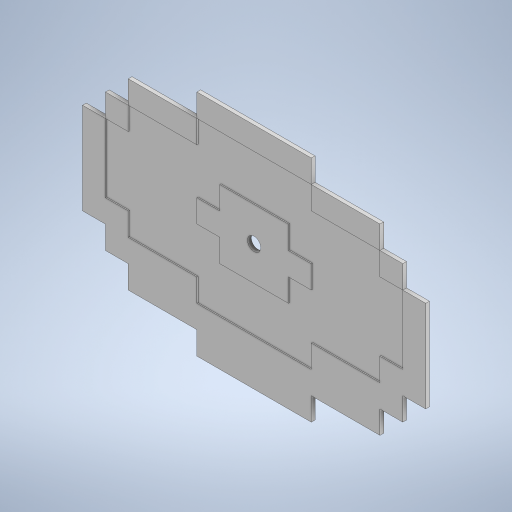
# Autodesk Inventor part: horizantal cut norm center
Saved by Autodesk Inventor 2024 (Build 280153000, 153)
## iProperties
Created: 2024-02-02
Part Number: horizantal cut norm center
Material: Generic
Document SubType Name: Modeling
Designer: newic
Density: 1 g/cm^3
Appearance: Default
Author: newic
Autodesk Inventor part; units mm, degrees
ref_plane "YZ Plane" through (0, 0, 0) normal (1, 0, 0) x (0, 1, 0)
ref_plane "XZ Plane" through (0, 0, 0) normal (0, 1, 0) x (-1, 0, 0)
ref_plane "XY Plane" through (0, 0, 0) normal (0, 0, 1) x (1, 0, 0)
sketch "Sketch1" plane through (0, 0, 0) normal (0, 0, 1) x (1, 0, 0)
  circle A0 centre (0, 0) radius 152.4
  circle A1 centre (0, 0) radius 5.5
  dimension "d0" = 304.8
  dimension "d1" = 11
  constraints: 2 centre point, 2 coincident
  measures "d0" diameter of A0
  measures "d1" diameter of A1
extrude "Extrusion1" add sketch "Sketch1" along normal blind 2.2
fillet "Fillet1" radius 1.1 2 edges at (-152.4, 0, 0) (-152.4, 0, 2.2)
sketch "Sketch2" plane through (0, 0, 2.2) normal (0, 0, 1) x (1, 0, 0)
  line L0 (206.2137, 42.4617) -> (289.822, 42.4617) construction
  line L1 (289.822, 42.4617) -> (289.822, -13.3654) construction
  line L2 (289.822, -13.3654) -> (206.2137, -13.3654) construction
  line L3 (206.2137, -13.3654) -> (206.2137, 42.4617) construction
  line L4 (9.525, 9.525) -> (-9.525, 9.525)
  line L5 (-9.525, 9.525) -> (-9.525, -9.525)
  line L6 (-9.525, -9.525) -> (9.525, -9.525)
  line L7 (9.525, -9.525) -> (9.525, 9.525)
  line L8 (-123.825, 28.575) -> (-104.775, 28.575)
  line L9 (-85.725, 28.575) -> (-66.675, 28.575)
  line L10 (-85.725, 28.575) -> (-104.775, 28.575)
  line L11 (-9.525, 28.575) -> (-28.575, 28.575)
  line L12 (-47.625, 28.575) -> (-28.575, 28.575)
  line L13 (-47.625, 28.575) -> (-66.675, 28.575)
  line L14 (-9.525, 9.525) -> (-9.525, 28.575)
  line L15 (-9.525, 28.575) -> (9.525, 28.575)
  line L16 (9.525, 28.575) -> (9.525, 9.525)
  line L17 (-9.525, -28.575) -> (-9.525, -9.525)
  line L18 (9.525, -9.525) -> (9.525, -28.575)
  line L19 (-123.825, -47.625) -> (-142.875, -47.625)
  line L20 (-123.825, -47.625) -> (-104.775, -47.625)
  line L21 (-85.725, -47.625) -> (-104.775, -47.625)
  line L22 (-85.725, -47.625) -> (-66.675, -47.625)
  line L23 (-47.625, -47.625) -> (-66.675, -47.625)
  line L24 (-47.625, -47.625) -> (-28.575, -47.625)
  line L25 (-9.525, -47.625) -> (-28.575, -47.625)
  line L26 (-9.525, -28.575) -> (-9.525, -47.625)
  line L27 (9.525, -47.625) -> (9.525, -28.575)
  line L28 (142.875, 28.575) -> (123.825, 28.575)
  line L29 (104.775, 28.575) -> (123.825, 28.575)
  line L30 (104.775, 28.575) -> (85.725, 28.575)
  line L31 (66.675, 28.575) -> (85.725, 28.575)
  line L32 (66.675, 28.575) -> (47.625, 28.575)
  line L33 (28.575, 28.575) -> (47.625, 28.575)
  line L34 (28.575, 28.575) -> (9.525, 28.575)
  line L35 (104.775, -47.625) -> (123.825, -47.625)
  line L36 (104.775, -47.625) -> (85.725, -47.625)
  line L37 (142.875, -47.625) -> (123.825, -47.625)
  line L38 (66.675, -47.625) -> (85.725, -47.625)
  line L39 (66.675, -47.625) -> (47.625, -47.625)
  line L40 (28.575, -47.625) -> (47.625, -47.625)
  line L41 (28.575, -47.625) -> (9.525, -47.625)
  line L42 (0, 9.525) -> (0, -9.525)
  line L43 (-9.525, 0) -> (9.525, 0)
  line L44 (0, 0) -> (-4.1012, 3.8959)
  line L45 (-142.875, 28.575) -> (-123.825, 28.575)
  line L46 (-123.825, 28.575) -> (-123.825, 9.525)
  line L47 (-123.825, 9.525) -> (-142.875, 9.525)
  line L48 (-142.875, 9.525) -> (-142.875, 28.575)
  line L49 (-142.875, -9.525) -> (-123.825, -9.525)
  line L50 (-123.825, -9.525) -> (-123.825, 9.525)
  line L51 (-142.875, 9.525) -> (-142.875, -9.525)
  line L52 (-123.825, -47.625) -> (-123.825, -28.575)
  line L53 (-123.825, -28.575) -> (-142.875, -28.575)
  line L54 (-142.875, -28.575) -> (-142.875, -47.625)
  line L55 (-123.825, -9.525) -> (-123.825, -28.575)
  line L56 (-142.875, -28.575) -> (-142.875, -9.525)
  line L57 (123.825, -47.625) -> (142.875, -47.625)
  line L58 (142.875, 28.575) -> (123.825, 28.575)
  line L59 (123.825, 28.575) -> (123.825, 9.525)
  line L60 (123.825, 9.525) -> (142.875, 9.525)
  line L61 (142.875, 9.525) -> (142.875, 28.575)
  line L62 (123.825, -9.525) -> (123.825, 9.525)
  line L63 (142.875, -9.525) -> (123.825, -9.525)
  line L64 (142.875, 9.525) -> (142.875, -9.525)
  line L65 (123.825, -9.525) -> (123.825, -28.575)
  line L66 (123.825, -47.625) -> (123.825, -28.575)
  line L67 (142.875, -28.575) -> (142.875, -9.525)
  line L68 (123.825, -28.575) -> (142.875, -28.575)
  line L69 (142.875, -28.575) -> (142.875, -47.625)
  line L70 (-123.825, 28.575) -> (-104.775, 28.575)
  line L71 (-104.775, 28.575) -> (-104.775, 47.625)
  line L72 (-104.775, 47.625) -> (-123.825, 47.625)
  line L73 (-123.825, 47.625) -> (-123.825, 28.575)
  line L74 (123.825, 28.575) -> (104.775, 28.575)
  line L75 (104.775, 28.575) -> (104.775, 47.625)
  line L76 (104.775, 47.625) -> (123.825, 47.625)
  line L77 (123.825, 47.625) -> (123.825, 28.575)
  line L78 (123.825, -47.625) -> (104.775, -47.625)
  line L79 (104.775, -47.625) -> (104.775, -66.675)
  line L80 (104.775, -66.675) -> (123.825, -66.675)
  line L81 (123.825, -66.675) -> (123.825, -47.625)
  line L82 (-123.825, -47.625) -> (-104.775, -47.625)
  line L83 (-104.775, -47.625) -> (-104.775, -66.675)
  line L84 (-104.775, -66.675) -> (-123.825, -66.675)
  line L85 (-123.825, -66.675) -> (-123.825, -47.625)
  line L86 (104.775, -66.675) -> (85.725, -66.675)
  line L87 (85.725, -66.675) -> (85.725, -85.725)
  line L88 (85.725, -85.725) -> (104.775, -85.725)
  line L89 (104.775, -85.725) -> (104.775, -66.675)
  line L90 (-104.775, -66.675) -> (-85.725, -66.675)
  line L91 (-85.725, -66.675) -> (-85.725, -85.725)
  line L92 (-85.725, -85.725) -> (-104.775, -85.725)
  line L93 (-104.775, -85.725) -> (-104.775, -66.675)
  line L94 (-66.675, -66.675) -> (-85.725, -66.675)
  line L95 (-85.725, -85.725) -> (-66.675, -85.725)
  line L96 (-66.675, -85.725) -> (-66.675, -66.675)
  line L97 (-47.625, -66.675) -> (-47.625, -85.725)
  line L98 (-47.625, -85.725) -> (-66.675, -85.725)
  line L99 (-66.675, -66.675) -> (-47.625, -66.675)
  line L100 (66.675, -66.675) -> (85.725, -66.675)
  line L101 (85.725, -85.725) -> (66.675, -85.725)
  line L102 (66.675, -85.725) -> (66.675, -66.675)
  line L103 (47.625, -66.675) -> (47.625, -85.725)
  line L104 (66.675, -66.675) -> (47.625, -66.675)
  line L105 (47.625, -85.725) -> (66.675, -85.725)
  line L106 (-47.625, -85.725) -> (-28.575, -85.725)
  line L107 (-28.575, -85.725) -> (-28.575, -104.775)
  line L108 (-28.575, -104.775) -> (-47.625, -104.775)
  line L109 (-47.625, -104.775) -> (-47.625, -85.725)
  line L110 (-9.525, -85.725) -> (-28.575, -85.725)
  line L111 (-28.575, -104.775) -> (-9.525, -104.775)
  line L112 (-9.525, -104.775) -> (-9.525, -85.725)
  line L113 (28.575, -85.725) -> (9.525, -85.725)
  line L114 (9.525, -85.725) -> (9.525, -104.775)
  line L115 (9.525, -104.775) -> (28.575, -104.775)
  line L116 (28.575, -104.775) -> (28.575, -85.725)
  line L117 (-9.525, -85.725) -> (9.525, -85.725)
  line L118 (9.525, -104.775) -> (-9.525, -104.775)
  line L119 (28.575, -85.725) -> (47.625, -85.725)
  line L120 (47.625, -85.725) -> (47.625, -104.775)
  line L121 (47.625, -104.775) -> (28.575, -104.775)
  line L122 (-104.775, 47.625) -> (-85.725, 47.625)
  line L123 (-85.725, 47.625) -> (-85.725, 66.675)
  line L124 (-85.725, 66.675) -> (-104.775, 66.675)
  line L125 (-104.775, 66.675) -> (-104.775, 47.625)
  line L126 (104.775, 47.625) -> (85.725, 47.625)
  line L127 (85.725, 47.625) -> (85.725, 66.675)
  line L128 (85.725, 66.675) -> (104.775, 66.675)
  line L129 (104.775, 66.675) -> (104.775, 47.625)
  line L130 (-66.675, 47.625) -> (-85.725, 47.625)
  line L131 (-85.725, 66.675) -> (-66.675, 66.675)
  line L132 (-66.675, 66.675) -> (-66.675, 47.625)
  line L133 (-47.625, 47.625) -> (-47.625, 66.675)
  line L134 (-66.675, 47.625) -> (-47.625, 47.625)
  line L135 (-47.625, 66.675) -> (-66.675, 66.675)
  line L136 (66.675, 47.625) -> (85.725, 47.625)
  line L137 (85.725, 66.675) -> (66.675, 66.675)
  line L138 (66.675, 66.675) -> (66.675, 47.625)
  line L139 (47.625, 47.625) -> (47.625, 66.675)
  line L140 (66.675, 47.625) -> (47.625, 47.625)
  line L141 (47.625, 66.675) -> (66.675, 66.675)
  line L142 (-47.625, 66.675) -> (-28.575, 66.675)
  line L143 (-28.575, 66.675) -> (-28.575, 85.725)
  line L144 (-28.575, 85.725) -> (-47.625, 85.725)
  line L145 (-47.625, 85.725) -> (-47.625, 66.675)
  line L146 (47.625, 66.675) -> (28.575, 66.675)
  line L147 (28.575, 66.675) -> (28.575, 85.725)
  line L148 (28.575, 85.725) -> (47.625, 85.725)
  line L149 (47.625, 85.725) -> (47.625, 66.675)
  line L150 (-9.525, 66.675) -> (-28.575, 66.675)
  line L151 (-28.575, 85.725) -> (-9.525, 85.725)
  line L152 (-9.525, 85.725) -> (-9.525, 66.675)
  line L153 (28.575, 66.675) -> (9.525, 66.675)
  line L154 (9.525, 66.675) -> (9.525, 85.725)
  line L155 (9.525, 85.725) -> (28.575, 85.725)
  line L156 (28.575, 85.725) -> (28.575, 66.675)
  line L157 (-9.525, 66.675) -> (9.525, 66.675)
  line L158 (9.525, 85.725) -> (-9.525, 85.725)
  circle A0 centre (0, 0) radius 225.16
  point P0 (-123.825, -9.525)
  point P1 (-123.825, -47.625)
  point P2 (123.825, -9.525)
  dimension "d22" = 19.05
  dimension "d23" = 19.05
  dimension "d29" = 19.05
  dimension "d30" = 19.05
  dimension "d31" = 19.05
  dimension "d32" = 19.05
  dimension "d33" = 19.05
  dimension "d34" = 19.05
  dimension "d35" = 19.05
  dimension "d36" = 19.05
  dimension "d39" = 19.05
  dimension "d40" = 19.05
  dimension "d45" = 19.05
  dimension "d46" = 19.05
  dimension "d50" = 19.05
  dimension "d51" = 19.05
  dimension "d52" = 19.05
  dimension "d53" = 19.05
  dimension "d58" = 19.05
  dimension "d59" = 19.05
  dimension "d60" = 19.05
  dimension "d61" = 19.05
  constraints: 310 end point, 60 symmetric about line, 24 parallel, 12 horizontal, 12 perpendicular, 5 midpoint, 1 centre point, 1 coincident, 2 other
  measures "d22" distance of L46.end L47.end
  measures "d23" distance of L45.end L46.end
  measures "d29" distance of L72.end L71.end
  measures "d30" distance of L71.end L70.end
  measures "d31" distance of L75.end L76.end
  measures "d32" distance of L74.end L75.end
  measures "d33" distance of L80.end L79.end
  measures "d34" distance of L79.end L78.end
  measures "d35" distance of L83.end L84.end
  measures "d36" distance of L82.end L83.end
  measures "d39" distance of L91.end L92.end
  measures "d40" distance of L90.end L91.end
  measures "d45" distance of L107.end L108.end
  measures "d46" distance of L106.end L107.end
  measures "d50" distance of L124.end L123.end
  measures "d51" distance of L123.end L122.end
  measures "d52" distance of L127.end L128.end
  measures "d53" distance of L126.end L127.end
  measures "d58" distance of L144.end L143.end
  measures "d59" distance of L143.end L142.end
  measures "d60" distance of L147.end L148.end
  measures "d61" distance of L146.end L147.end
extrude "Extrusion2" cut sketch "Sketch2" against normal blind 25.4
sketch "Sketch3" plane through (0, 0, 2.2) normal (0, 0, 1) x (1, 0, 0)
  line L0 (194.8549, 38.1597) -> (278.4632, 38.1597) construction
  line L1 (278.4632, 38.1597) -> (278.4632, -17.6674) construction
  line L2 (278.4632, -17.6674) -> (194.8549, -17.6674) construction
  line L3 (194.8549, -17.6674) -> (194.8549, 38.1597) construction
  line L4 (-123.825, 28.575) -> (-104.775, 28.575)
  line L5 (-123.825, -47.625) -> (-142.875, -47.625)
  line L6 (104.775, 28.575) -> (123.825, 28.575)
  line L7 (142.875, 28.575) -> (123.825, 28.575)
  line L8 (142.875, -47.625) -> (123.825, -47.625)
  line L9 (-142.875, 28.575) -> (-123.825, 28.575)
  line L10 (-123.825, 28.575) -> (-123.825, 9.525)
  line L11 (-142.875, 9.525) -> (-142.875, 28.575)
  line L12 (-123.825, -9.525) -> (-123.825, 9.525)
  line L13 (-142.875, 9.525) -> (-142.875, -9.525)
  line L14 (-123.825, -9.525) -> (-123.825, -28.575)
  line L15 (-142.875, -28.575) -> (-142.875, -9.525)
  line L16 (-142.875, -28.575) -> (-142.875, -47.625)
  line L17 (123.825, -9.525) -> (123.825, 9.525)
  line L18 (142.875, 9.525) -> (142.875, -9.525)
  line L19 (123.825, 28.575) -> (123.825, 9.525)
  line L20 (142.875, 9.525) -> (142.875, 28.575)
  line L21 (142.875, 28.575) -> (123.825, 28.575)
  line L22 (123.825, -9.525) -> (123.825, -28.575)
  line L23 (142.875, -28.575) -> (142.875, -9.525)
  line L24 (142.875, -28.575) -> (142.875, -47.625)
  line L25 (123.825, -47.625) -> (142.875, -47.625)
  line L26 (-123.825, 28.575) -> (-104.775, 28.575)
  line L27 (-104.775, 28.575) -> (-104.775, 47.625)
  line L28 (-104.775, 47.625) -> (-123.825, 47.625)
  line L29 (-123.825, 47.625) -> (-123.825, 28.575)
  line L30 (123.825, 28.575) -> (104.775, 28.575)
  line L31 (104.775, 28.575) -> (104.775, 47.625)
  line L32 (104.775, 47.625) -> (123.825, 47.625)
  line L33 (123.825, 47.625) -> (123.825, 28.575)
  line L34 (104.775, -66.675) -> (123.825, -66.675)
  line L35 (123.825, -66.675) -> (123.825, -47.625)
  line L36 (-104.775, -66.675) -> (-123.825, -66.675)
  line L37 (-123.825, -66.675) -> (-123.825, -47.625)
  line L38 (85.725, -85.725) -> (104.775, -85.725)
  line L39 (104.775, -85.725) -> (104.775, -66.675)
  line L40 (-85.725, -85.725) -> (-104.775, -85.725)
  line L41 (-104.775, -85.725) -> (-104.775, -66.675)
  line L42 (-85.725, -85.725) -> (-66.675, -85.725)
  line L43 (-47.625, -85.725) -> (-66.675, -85.725)
  line L44 (85.725, -85.725) -> (66.675, -85.725)
  line L45 (47.625, -85.725) -> (66.675, -85.725)
  line L46 (-28.575, -104.775) -> (-47.625, -104.775)
  line L47 (-47.625, -104.775) -> (-47.625, -85.725)
  line L48 (-28.575, -104.775) -> (-9.525, -104.775)
  line L49 (9.525, -104.775) -> (-9.525, -104.775)
  line L50 (9.525, -104.775) -> (28.575, -104.775)
  line L51 (47.625, -85.725) -> (47.625, -104.775)
  line L52 (47.625, -104.775) -> (28.575, -104.775)
  line L53 (-104.775, 47.625) -> (-85.725, 47.625)
  line L54 (-85.725, 66.675) -> (-104.775, 66.675)
  line L55 (-104.775, 66.675) -> (-104.775, 47.625)
  line L56 (104.775, 66.675) -> (104.775, 47.625)
  line L57 (-66.675, 47.625) -> (-85.725, 47.625)
  line L58 (-85.725, 66.675) -> (-66.675, 66.675)
  line L59 (-66.675, 47.625) -> (-47.625, 47.625)
  line L60 (-47.625, 66.675) -> (-66.675, 66.675)
  line L61 (-47.625, 47.625) -> (-47.625, 66.675)
  line L62 (-47.625, 85.725) -> (-47.625, 66.675)
  circle A0 centre (0, 0) radius 225.16
  line L63 (-47.625, 85.725) -> (47.625, 85.725)
  line L64 (47.625, 85.725) -> (47.625, 66.675)
  line L65 (47.625, 66.675) -> (-47.625, 66.675)
  line L66 (-47.625, 66.675) -> (-47.625, 85.725)
  line L67 (47.625, 66.675) -> (104.775, 66.675)
  line L68 (104.775, 66.675) -> (104.775, 47.625)
  line L69 (104.775, 47.625) -> (47.625, 47.625)
  line L70 (47.625, 47.625) -> (47.625, 66.675)
  line L71 (-123.825, -28.575) -> (-104.775, -28.575)
  line L72 (-104.775, -28.575) -> (-104.775, -47.625)
  line L73 (-104.775, -47.625) -> (-85.725, -47.625)
  line L74 (-85.725, -47.625) -> (-47.625, -47.625)
  line L75 (-47.625, -47.625) -> (-47.625, -66.675)
  line L76 (-47.625, -66.675) -> (47.625, -66.675)
  line L77 (104.775, -47.625) -> (47.625, -47.625)
  line L78 (47.625, -47.625) -> (47.625, -66.675)
  line L79 (123.825, -28.575) -> (104.775, -28.575)
  line L80 (104.775, -28.575) -> (104.775, -47.625)
  line L81 (9.525, -28.575) -> (-9.525, -28.575)
  line L82 (28.575, -9.525) -> (28.575, -28.575)
  line L83 (28.575, -28.575) -> (9.525, -28.575)
  line L84 (-28.575, -9.525) -> (-28.575, -28.575)
  line L85 (-28.575, -28.575) -> (-9.525, -28.575)
  line L86 (-9.525, 28.575) -> (-28.575, 28.575)
  line L87 (-28.575, 28.575) -> (-28.575, 9.525)
  line L88 (-9.525, 28.575) -> (9.525, 28.575)
  line L89 (9.525, 28.575) -> (28.575, 28.575)
  line L90 (28.575, 28.575) -> (28.575, 9.525)
  line L91 (28.575, 9.525) -> (47.625, 9.525)
  line L92 (47.625, 9.525) -> (47.625, -9.525)
  line L93 (47.625, -9.525) -> (28.575, -9.525)
  line L94 (-28.575, 9.525) -> (-47.625, 9.525)
  line L95 (-47.625, 9.525) -> (-47.625, -9.525)
  line L96 (-47.625, -9.525) -> (-28.575, -9.525)
  circle A1 centre (0, 0) radius 5.5
  point P0 (-123.825, -9.525)
  point P1 (-123.825, -47.625)
  point P2 (123.825, -9.525)
  point P3 (112.4662, 24.273)
  point P4 (112.4662, -51.927)
  point P5 (-135.1838, -51.927)
  dimension "d94" = 19.05
  dimension "d96" = 19.05
  dimension "d97" = 19.05
  dimension "d98" = 19.05
  dimension "d99" = 19.05
  dimension "d100" = 19.05
  dimension "d102" = 19.05
  dimension "d103" = 19.05
  dimension "d104" = 19.05
  dimension "d105" = 19.05
  constraints: 186 end point, 16 horizontal, 12 parallel, 12 perpendicular, 2 centre point, 1 coincident, 2 other
  measures "d94" distance of L81.start L81.end
  measures "d96" distance of L82.end L83.end
  measures "d97" distance of L82.start L82.end
  measures "d98" distance of L85.end L84.end
  measures "d99" distance of L84.end L84.start
  measures "d100" distance of L86.end L86.start
  measures "d102" distance of L92.end L93.end
  measures "d103" distance of L91.end L92.end
  measures "d104" distance of L96.end L95.end
  measures "d105" distance of L95.end L94.end
extrude "Extrusion3" add sketch "Sketch3" along normal blind 0.9 contours L29 L28 L27 L4 | L10 L12 L14 L71 L72 L73 L74 L75 L76 L78 L77 L80 L79 L22 L17 L19 L7 L20 L18 L23 L24 L8 L35 L34 L39 L38 L44 L45 L51 L52 L50 L49 L48 L46 L47 L43 L42 L40 L41 L36 L37 L5 L16 L15 L13 L11 L9 | L55 L54 L58 L60 L61 L59 L57 L53 | L62 L63 L64 L65 | L67 L56 L69 L70 | L32 L33 L6 L31 | L81 L85 L84 L96 L95 L94 L87 L86 L88 L89 L90 L91 L92 L93 L82 L83
body "Solid1"
